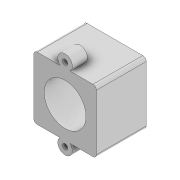
# Autodesk Inventor part: 00_CCTV_M12_VCM_large
Saved by Autodesk Inventor 2022 (Build 260153000, 153)
## iProperties
Created: 2022-07-18
Part Number: 00_CCTV_M12_VCM_large
Material: Generisch
Document SubType Name: Modeling
Designer: diederichbenedict
Density: 1 g/cm^3
Appearance: Vorgabe
Author: diederichbenedict
Autodesk Inventor part; units mm, degrees
ref_plane "YZ Plane" through (0, 0, 0) normal (1, 0, 0) x (0, 1, 0)
ref_plane "XZ Plane" through (0, 0, 0) normal (0, 1, 0) x (-1, 0, 0)
ref_plane "XY Plane" through (0, 0, 0) normal (0, 0, 1) x (1, 0, 0)
sketch "Skizze1" plane through (0, 0, 0) normal (0, 0, 1) x (1, 0, 0)
  line L0 (9, -9) -> (-9, -9)
  line L1 (-9, -9) -> (-9, 9)
  line L2 (-9, 9) -> (9, 9)
  line L3 (9, 9) -> (9, -9)
  line L4 (9, -9) -> (-9, 9) construction
  line L5 (-9, -9) -> (9, 9) construction
  circle A0 centre (0, 0) radius 6
  dimension "d0" = 18
  dimension "d1" = 18
  dimension "d2" = 12
  constraints: 12 end point, 2 midpoint, 2 parallel, 1 centre point, 1 coincident, 1 horizontal, 1 perpendicular
  measures "d0" distance of L1.end L2.end
  measures "d1" distance of L0.end L1.end
  measures "d2" diameter of A0
extrude "Extrusion1" add sketch "Skizze1" along normal blind 10
fillet "Rundung1" radius 1 4 edges at (9, 9, 5) (-9, 9, 5) (9, -9, 5) (-9, -9, 5)
sketch "Skizze2" plane through (0, 0, 10) normal (0, 0, 1) x (1, 0, 0)
  arc A0 (-9, -8) -> (-8, -9) centre (-8, -8) ccw projected
  line L0 (-8, -9) -> (8, -9) projected
  arc A1 (8, -9) -> (9, -8) centre (8, -8) ccw projected
  line L1 (9, -8) -> (9, 8) projected
  arc A2 (9, 8) -> (8, 9) centre (8, 8) ccw projected
  line L2 (8, 9) -> (-8, 9) projected
  arc A3 (-8, 9) -> (-9, 8) centre (-8, 8) ccw projected
  line L3 (-9, 8) -> (-9, -8) projected
  circle A4 centre (0, 0) radius 6 projected
  circle A5 centre (0, 10.5) radius 0.75
  circle A6 centre (0, -10.5) radius 0.75
  circle A7 centre (0, 10.5) radius 2.1
  circle A8 centre (0, -10.5) radius 2.1
  point P0 (-1.4697, -9)
  point P1 (1.4697, -9)
  point P2 (1.4697, 9)
  point P3 (-1.4697, 9)
  dimension "d6" = 1.5
  dimension "d7" = 1.5
  dimension "d8" = 10.5
  dimension "d9" = 10.5
  dimension "d10" = 4.2
  dimension "d11" = 4.2
  constraints: 4 centre point, 2 coincident
  measures "d6" diameter of A5
  measures "d7" diameter of A6
  measures "d8" distance of A5.centre point (0, 0)
  measures "d9" distance of A6.centre point (0, 0)
  measures "d10" diameter of A7
  measures "d11" diameter of A8
extrude "Extrusion2" add sketch "Skizze2" along normal blind 4.3
